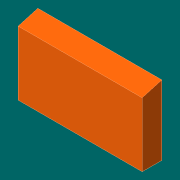
# Autodesk Inventor part: mirrorSuppourt
Saved by Autodesk Inventor 2016 (Build 200138000, 138)
## iProperties
Created: 2015-10-14
Part Number: mirrorSuppourt
Material: PC/ABS Plastic
Document SubType Name: Modeling
Designer: Sawaiz
Density: 0.357273 g/cm^3
Appearance: Smooth - Light Orange
Author: Sawaiz
Autodesk Inventor part; units mm, degrees
ref_plane "YZ Plane" through (0, 0, 0) normal (1, 0, 0) x (0, 1, 0)
ref_plane "XZ Plane" through (0, 0, 0) normal (0, 1, 0) x (-1, 0, 0)
ref_plane "XY Plane" through (0, 0, 0) normal (0, 0, 1) x (1, 0, 0)
sketch "Sketch1" plane through (0, 0, 0) normal (0, 1, 0) x (-1, 0, 0)
  line L0 (0, 0) -> (78.376, 22.474)
  line L1 (78.376, 22.474) -> (78.376, 0)
  line L2 (78.376, 0) -> (72.026, 0)
  line L3 (72.026, 0) -> (72.026, 20.6531)
  line L4 (0, 0) -> (50.5854, 0)
  dimension "d0" = 6.35
  dimension "d1" = 16
  dimension "d2" = 78.376
  constraints: 10 end point, 2 perpendicular, 1 collinear, 1 horizontal, 1 point on line, 1 vertical
  measures "d0" distance between parallel lines of L1 L3
  measures "d1" angle of L2 L0
  measures "d2" distance from line of L0.start L1
extrude "Extrusion1" add sketch "Sketch1" along normal mid plane 40
equation "\"d0\" = acrylicThickness"
equation "\"d1\" = mirrorAngle"
equation "\"d2\" = -centerThickness + depth - aerogelThickness - fresnelThickness"
equation "\"d3\" = mirrorSuppourtWidth"
equation "\"acrylicThickness\" = 6.35"
equation "\"aerogelThickness\" = 20"
equation "\"depth\" = 100"
equation "\"mirrorAngle\" = 16deg"
equation "\"detectorWidth\" = 52"
equation "\"detectorHeight\" = 52"
equation "\"mirrorThickness\" = 3"
equation "\"fresnelThickness\" = 0.1"
equation "\"focalLength\" = 76.2"
equation "\"ior\" = 1.49"
equation "\"centerThickness\" = 1.524"
equation "\"fresnelAngle\" = 90deg"
equation "\"fresnelEffectiveDiameter\" = 76.2"
equation "\"mirrorSuppourtWidth\" = 40"
body "Solid1"
